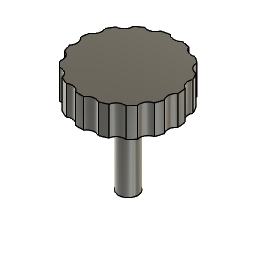
ButtonExtander (Autodesk Fusion 360 design; units mm, degrees)
Autodesk Fusion 360 part; units mm, degrees
sketch "Sketch5" plane through (0, 0, 0) normal (0, 0, -1) x (1, 0, 0)
  arc A0 (12.9762, -21.3686) -> (7.1972, -23.9416) centre (11.3886, -25.5793) ccw
  arc A1 (12.9762, -21.3686) -> (16.3129, -18.9444) centre (0, 0) ccw
  arc A2 (20.5458, -14.2433) -> (16.3129, -18.9444) centre (20.8081, -18.7357) ccw
  arc A3 (20.5458, -14.2433) -> (22.6079, -10.6715) centre (0, 0) ccw
  arc A4 (24.5628, -4.6552) -> (22.6079, -10.6715) centre (26.6296, -8.6525) ccw
  arc A5 (24.5628, -4.6552) -> (24.9939, -0.5534) centre (0, 0) ccw
  arc A6 (24.3326, 5.7378) -> (24.9939, -0.5534) centre (27.8466, 2.9268) ccw
  arc A7 (24.3326, 5.7378) -> (23.0581, 9.6604) centre (0, 0) ccw
  arc A8 (19.8952, 15.1388) -> (23.0581, 9.6604) centre (24.2487, 14) ccw
  arc A9 (19.8952, 15.1388) -> (17.1354, 18.2038) centre (0, 0) ccw
  arc A10 (12.0177, 21.922) -> (17.1354, 18.2038) centre (16.458, 22.6525) ccw
  arc A11 (12.0177, 21.922) -> (8.2499, 23.5996) centre (0, 0) ccw
  arc A12 (2.0622, 24.9148) -> (8.2499, 23.5996) centre (5.8215, 27.3881) ccw
  arc A13 (2.0622, 24.9148) -> (-2.0622, 24.9148) centre (0, 0) ccw
  arc A14 (-8.2499, 23.5996) -> (-2.0622, 24.9148) centre (-5.8215, 27.3881) ccw
  arc A15 (-8.2499, 23.5996) -> (-12.0177, 21.922) centre (0, 0) ccw
  arc A16 (-17.1354, 18.2038) -> (-12.0177, 21.922) centre (-16.458, 22.6525) ccw
  arc A17 (-17.1354, 18.2038) -> (-19.8952, 15.1388) centre (0, 0) ccw
  arc A18 (-23.0581, 9.6604) -> (-19.8952, 15.1388) centre (-24.2487, 14) ccw
  arc A19 (-23.0581, 9.6604) -> (-24.3326, 5.7378) centre (0, 0) ccw
  arc A20 (-24.9939, -0.5534) -> (-24.3326, 5.7378) centre (-27.8466, 2.9268) ccw
  arc A21 (-24.9939, -0.5534) -> (-24.5628, -4.6552) centre (0, 0) ccw
  arc A22 (-22.6079, -10.6715) -> (-24.5628, -4.6552) centre (-26.6296, -8.6525) ccw
  arc A23 (-22.6079, -10.6715) -> (-20.5458, -14.2433) centre (0, 0) ccw
  arc A24 (-16.3129, -18.9444) -> (-20.5458, -14.2433) centre (-20.8081, -18.7357) ccw
  arc A25 (-16.3129, -18.9444) -> (-12.9762, -21.3686) centre (0, 0) ccw
  arc A26 (-7.1972, -23.9416) -> (-12.9762, -21.3686) centre (-11.3886, -25.5793) ccw
  arc A27 (-7.1972, -23.9416) -> (-3.163, -24.7991) centre (0, 0) ccw
  arc A28 (3.163, -24.7991) -> (-3.163, -24.7991) centre (0, -28) ccw
  arc A29 (3.163, -24.7991) -> (7.1972, -23.9416) centre (0, 0) ccw
  circle A30 centre (0, 0) radius 5
  circle A31 centre (0, 0) radius 3.25
  line L0 (-2.0767, 2.5) -> (-2.0767, -2.5)
  dimension "d3" = 10
  dimension "d4" = 6.5
  dimension "d5" = 5
  constraint concentric A1 A30
  constraint concentric A1 A31
  constraint coincident A31 L0.start
  constraint coincident A31 L0.end
  constraint vertical L0
  measures "d3" diameter of A30
  measures "d4" diameter of A31
  measures "d5" distance of L0.start L0.end
sketch "Sketch1" plane through (0, 0, 0) normal (0, 0, 1) x (1, 0, 0)
  circle A0 centre (0, 0) radius 25
  constraint coincident A0.centre origin
extrude "Extrude1" add sketch "Sketch1" along normal blind 15
sketch "Sketch4" plane through (0, 0, 15) normal (0, 0, 1) x (-1, 0, 0)
  circle A0 centre (0, 0) radius 25
  circle A1 centre (0, -28) radius 4.5
  dimension "d24" = 9
  measures "d24" diameter of A1
extrude "Extrude3" cut sketch "Sketch4" against normal up to surface (15 mm away) contours A0 A1 picked at (-0.1062, -24.4889)
pattern_circular "C-Pattern1" count 15 over 360 about axis through (0, 0, 1.75) along (0, 0, 1) of "Extrude3"
extrude "Extrude5" add sketch "Sketch5" along normal blind 40 contours A30 | A31 L0 picked at (-2.6499, -0.3124)
